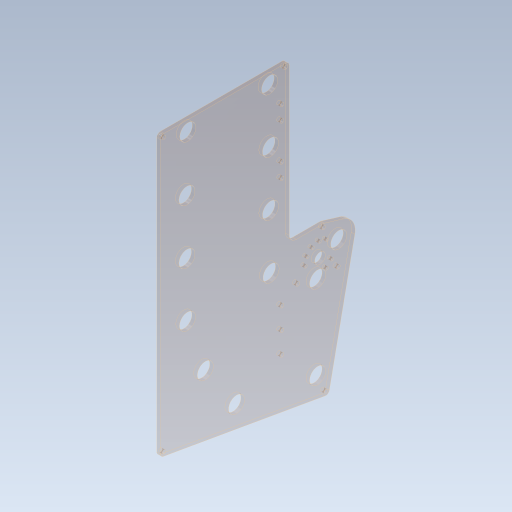
# Autodesk Inventor part: sketchers
Saved by Autodesk Inventor 2024 (Build 280153000, 153)
## iProperties
Created: 2024-07-27
Part Number: sketchers
Material: Polycarbonate, Smoke
Document SubType Name: Modeling
Designer: Oscar
Density: 1.2 g/cm^3
Appearance: Polycarbonate - Smoked
Author: Oscar
Autodesk Inventor part; units mm, degrees
ref_plane "YZ Plane" through (0, 0, 0) normal (1, 0, 0) x (0, 1, 0)
ref_plane "XZ Plane" through (0, 0, 0) normal (0, 1, 0) x (-1, 0, 0)
ref_plane "XY Plane" through (0, 0, 0) normal (0, 0, 1) x (1, 0, 0)
sketch "Sketch1" plane through (0, 0, 0) normal (1, 0, 0) x (0, 1, 0)
  line L0 (95.25, 812.8) -> (44.45, 812.8) construction
  line L1 (44.45, 812.8) -> (44.45, 0) construction
  line L2 (44.45, 0) -> (95.25, 0) construction
  line L3 (95.25, 0) -> (95.25, 812.8) construction
  line L4 (95.25, 0) -> (44.45, 0) construction
  line L5 (44.45, 0) -> (44.45, 25.4) construction
  line L6 (44.45, 25.4) -> (95.25, 25.4) construction
  line L7 (95.25, 25.4) -> (95.25, 0) construction
  circle A0 centre (190.5, 0) radius 50.8 construction
  circle A1 centre (95.25, 279.4) radius 25.4 construction
  circle A2 centre (274.6634, 275.1936) radius 9.525
  circle A3 centre (274.6634, 275.1936) radius 25.4 construction
  circle A4 centre (274.6634, 275.1936) radius 31.75 construction
  circle A5 centre (300.0634, 275.1936) radius 2.4892
  circle A6 centre (296.6604, 287.8936) radius 2.4892
  circle A7 centre (287.3634, 297.1907) radius 2.4892
  circle A8 centre (274.6634, 300.5936) radius 2.4892
  circle A9 centre (261.9634, 297.1907) radius 2.4892 construction
  circle A10 centre (252.6663, 287.8936) radius 2.4892 construction
  circle A11 centre (249.2634, 275.1936) radius 2.4892 construction
  circle A12 centre (252.6663, 262.4936) radius 2.4892
  circle A13 centre (261.9634, 253.1966) radius 2.4892
  circle A14 centre (274.6634, 249.7936) radius 2.4892 construction
  circle A15 centre (287.3634, 253.1966) radius 2.4892 construction
  circle A16 centre (296.6604, 262.4936) radius 2.4892
  circle A17 centre (609.6, 438.15) radius 50.8 construction
  circle A18 centre (274.6634, 275.1936) radius 30.48 construction
  circle A19 centre (587.8333, 365.125) radius 25.4 construction
  circle A20 centre (587.8333, 511.175) radius 25.4 construction
  line L8 (587.8333, 485.775) -> (587.8333, 390.525) construction
  circle A21 centre (490.3356, 512.7625) radius 14.351
  circle A22 centre (392.825, 512.7625) radius 14.351
  circle A23 centre (490.3356, 363.5375) radius 14.351
  line L9 (587.8333, 511.175) -> (490.3356, 512.7625) construction
  line L10 (587.8333, 365.125) -> (490.3356, 363.5375) construction
  circle A24 centre (490.3356, 512.7625) radius 25.4 construction
  circle A25 centre (490.3356, 363.5375) radius 25.4 construction
  line L11 (490.3356, 487.3625) -> (490.3356, 388.9375) construction
  circle A26 centre (392.825, 512.7625) radius 25.4 construction
  circle A27 centre (392.825, 363.5375) radius 25.4 construction
  circle A28 centre (392.825, 363.5375) radius 14.351
  line L12 (490.3356, 512.7625) -> (392.825, 512.7625) construction
  line L13 (490.3356, 363.5375) -> (392.825, 363.5375) construction
  line L14 (392.825, 487.3625) -> (392.825, 388.9375) construction
  circle A29 centre (295.3189, 511.8309) radius 25.4 construction
  circle A30 centre (295.3189, 362.6059) radius 25.4 construction
  circle A31 centre (203.1597, 479.9719) radius 25.4 construction
  circle A32 centre (295.3189, 511.8309) radius 14.351
  circle A33 centre (295.3189, 362.6059) radius 14.351
  circle A34 centre (203.1597, 479.9719) radius 14.351
  line L15 (392.825, 512.7625) -> (295.3189, 511.8309) construction
  line L16 (392.825, 363.5375) -> (295.3189, 362.6059) construction
  line L17 (295.3189, 486.4309) -> (295.3189, 388.0059) construction
  line L18 (295.3189, 511.8309) -> (203.1597, 479.9719) construction
  circle A35 centre (123.1487, 424.2353) radius 25.4 construction
  circle A36 centre (123.1487, 424.2353) radius 14.351
  line L19 (203.1597, 479.9719) -> (123.1487, 424.2353) construction
  circle A37 centre (95.25, 279.4) radius 14.351
  line L20 (609.6, 355.6) -> (44.45, 355.6) construction
  line L21 (44.45, 355.6) -> (44.45, 330.2) construction
  line L22 (44.45, 330.2) -> (609.6, 330.2) construction
  line L23 (609.6, 330.2) -> (609.6, 355.6) construction
  line L24 (95.25, 241.3) -> (44.45, 241.3) construction
  line L25 (44.45, 241.3) -> (44.45, 215.9) construction
  line L26 (44.45, 215.9) -> (95.25, 215.9) construction
  line L27 (95.25, 215.9) -> (95.25, 241.3) construction
  circle A38 centre (244.475, 279.4) radius 25.4 construction
  circle A39 centre (244.475, 279.4) radius 14.351
  line L28 (218.8463, 459.9947) -> (279.6322, 382.5831) construction
  circle A40 centre (274.6634, 275.1936) radius 8.89 construction
  circle A41 centre (286.5635, 241.6839) radius 26.67 construction
  circle A42 centre (244.475, 279.4) radius 21.59 construction
  circle A43 centre (286.5635, 241.6839) radius 14.351
  circle A44 centre (587.8333, 511.175) radius 14.351
  circle A45 centre (587.8333, 365.125) radius 14.351
  line L29 (44.45, 624.136) -> (44.45, 649.536) construction
  line L30 (95.25, 647.7) -> (609.6, 647.7) construction
  line L31 (609.6, 647.7) -> (609.6, 622.3) construction
  line L32 (609.6, 622.3) -> (95.25, 622.3) construction
  line L33 (95.25, 622.3) -> (95.25, 647.7) construction
  circle A46 centre (600.5333, 553.7721) radius 3.2639
  circle A47 centre (600.5333, 553.7721) radius 6.35 construction
  circle A48 centre (600.5333, 336.55) radius 3.2639
  circle A49 centre (600.5333, 336.55) radius 6.35 construction
  circle A50 centre (114.3, 553.7721) radius 3.2639
  circle A51 centre (114.3, 553.7721) radius 6.35 construction
  line L34 (595.0904, 535.5162) -> (598.719, 547.6868) construction
  circle A52 centre (63.5, 264.8503) radius 3.2639
  circle A53 centre (63.5, 264.8503) radius 6.35 construction
  line L35 (337.6816, 330.2) -> (600.5333, 330.2)
  line L36 (313.4556, 344.8233) -> (322.5239, 335.932) construction
  circle A54 centre (286.5635, 241.6839) radius 29.21 construction
  circle A55 centre (244.475, 279.4) radius 24.13 construction
  line L37 (72.1591, 268.8184) -> (69.2727, 267.4957) construction
  line L38 (609.6, 342.9) -> (44.45, 342.9) construction
  circle A56 centre (286.5635, 241.6839) radius 19.05 construction
  line L39 (262.4454, 263.2965) -> (264.8099, 261.1776) construction
  circle A57 centre (318.6316, 268.667) radius 3.2639
  circle A58 centre (254.5405, 314.8279) radius 3.2639
  circle A59 centre (244.6596, 242.3976) radius 3.2639
  line L40 (95.25, 558.8) -> (44.45, 558.8) construction
  line L41 (44.45, 558.8) -> (44.45, 533.4) construction
  line L42 (44.45, 533.4) -> (95.25, 533.4) construction
  line L43 (95.25, 533.4) -> (95.25, 558.8) construction
  line L44 (114.3, 560.1221) -> (600.5333, 560.1221)
  line L45 (108.0459, 554.8717) -> (57.2459, 265.95)
  line L46 (280.6003, 213.0891) -> (62.2036, 258.6341)
  circle A60 centre (318.6316, 268.667) radius 6.35 construction
  circle A61 centre (254.5405, 314.8279) radius 6.35 construction
  circle A62 centre (244.6596, 242.3976) radius 6.35 construction
  arc A63 (114.3, 560.1221) -> (108.0459, 554.8717) centre (114.3, 553.7721) ccw
  arc A64 (57.2459, 265.95) -> (62.2036, 258.6341) centre (63.5, 264.8503) ccw
  line L47 (312.3504, 269.5994) -> (306.0692, 270.5317) construction
  line L48 (313.7728, 264.5787) -> (308.914, 260.4903) construction
  line L49 (257.4152, 309.1658) -> (260.2899, 303.5038) construction
  line L50 (252.8051, 308.7196) -> (251.0697, 302.6114) construction
  line L51 (251.0087, 242.2895) -> (257.3577, 242.1814) construction
  line L52 (248.9458, 247.0828) -> (253.2321, 251.7679) construction
  line L53 (324.9816, 317.5) -> (324.9816, 268.667)
  arc A65 (337.6816, 330.2) -> (324.9816, 317.5) centre (337.6816, 317.5) ccw
  line L54 (324.7085, 266.8246) -> (314.5171, 233.2091)
  arc A66 (324.7085, 266.8246) -> (324.9816, 268.667) centre (318.6316, 268.667) ccw
  arc A67 (280.6003, 213.0891) -> (314.5171, 233.2091) centre (286.5635, 241.6839) ccw
  circle A68 centre (431.8, 342.9) radius 3.2639
  circle A69 centre (457.2, 342.9) radius 3.2639
  circle A70 centre (234.95, 342.9) radius 3.2639
  circle A71 centre (196.85, 342.9) radius 3.2639
  circle A72 centre (158.75, 342.9) radius 3.2639
  circle A73 centre (520.7, 342.9) radius 3.2639
  circle A74 centre (546.1, 342.9) radius 3.2639
  line L55 (606.8833, 553.7721) -> (606.8833, 336.55)
  arc A75 (606.8833, 553.7721) -> (600.5333, 560.1221) centre (600.5333, 553.7721) ccw
  arc A76 (600.5333, 330.2) -> (606.8833, 336.55) centre (600.5333, 336.55) ccw
  point P0 (0, 0)
  point P1 (273.4883, 247.5992)
  point P2 (276.276, 251.6898)
  point P3 (251.6966, 266.9984)
  point P4 (254.3358, 268.9733)
  dimension "d9" = 50.8
  dimension "d14" = 50.8
  dimension "d38" = 50.8
  dimension "d53" = 50.8
  dimension "d1" = 812.8
  dimension "d2" = 44.45
  dimension "d4" = 25.4
  dimension "d5" = 101.6
  dimension "d6" = 95.25
  dimension "d8" = 50.8
  dimension "d15" = 63.5
  dimension "d21" = 19.05
  dimension "d26" = 360
  dimension "d28" = 4.9784
  dimension "d29" = 438.15
  dimension "d30" = 514.35
  dimension "d36" = 60.96
  dimension "d39" = 50.8
  dimension "d41" = 95.25
  dimension "d45" = 28.702
  dimension "d47" = 97.5106
  dimension "d48" = 98.425
  dimension "d56" = 25.4
  dimension "d73" = 50.8
  dimension "d74" = 25.4
  dimension "d75" = 215.9
  dimension "d78" = 279.4
  dimension "d80" = 149.225
  dimension "d81" = 97.5106
  dimension "d82" = 147.4978
  dimension "d83" = 17.78
  dimension "d85" = 53.34
  dimension "d92" = 330.2
  dimension "d100" = 514.35
  dimension "d107" = 25.4
  dimension "d108" = 514.35
  dimension "d109" = 266.7
  dimension "d110" = 12.7
  dimension "d115" = 6.5278
  dimension "d116" = 12.7
  dimension "d122" = 2.54
  dimension "d123" = 2.54
  dimension "d128" = 3.175
  dimension "d133" = 38.1
  dimension "d134" = 3.175
  dimension "d135" = 194.9958
  dimension "d136" = 6.5278
  dimension "d137" = 25.4
  dimension "d138" = 533.4
  dimension "d139" = 19.05
  dimension "d140" = 19.05
  dimension "d141" = 12.7
  dimension "d142" = 6.35
  dimension "d143" = 12.7
  dimension "d144" = 43.18
  dimension "d149" = 25.4
  dimension "d151" = 6.5278
  dimension "d152" = 38.1
  dimension "d153" = 38.1
  dimension "d155" = 63.5
  dimension "d156" = 196.85
  dimension "d157" = 25.4
  dimension "d158" = 63.5
  dimension "d159" = 12.7
  constraints: 108 end point, 68 centre point, 47 point on circle, 32 point on line, 29 equal radius, 27 coincident, 20 tangent, 15 equal length, 11 parallel, 9 horizontal, 8 vertical alignment, 6 horizontal alignment, 6 perpendicular, 4 concentric, 4 vertical, 2 midpoint, 66 other
  measures "d1" distance of L1.end L0.end
  measures "d2" distance from line of point (0, 0) L1
  measures "d4" distance of L4.end L5.end
  measures "d5" diameter of A0
  measures "d15" diameter of A4
  measures "d21" diameter of A2
  measures "d28" diameter of A16
  measures "d29" distance from line of L2 point (609.6, 438.15)
  measures "d36" diameter of A18
  measures "d39" diameter of A20
  measures "d41" distance of L8.start L8.end
  measures "d45" diameter of A21
  measures "d47" distance of L9.start L9.end
  measures "d48" distance of L11.start L11.end
  measures "d56" distance of L22.end L20.start
  measures "d73" distance of L26.end L25.end
  measures "d74" distance of L25.end L24.end
  measures "d75" distance between parallel lines of L2 L26
  measures "d78" distance from line of L2 point (95.25, 279.4)
  measures "d80" distance of point (95.25, 279.4) A38.centre
  measures "d81" distance of A38.centre A30.centre
  measures "d82" distance of point (95.25, 279.4) A35.centre
  measures "d83" diameter of A40
  measures "d85" diameter of A41
  measures "d92" distance between parallel lines of L2 L22
  measures "d107" distance between parallel lines of L32 L30
  measures "d108" distance of L31.end L32.end
  measures "d109" distance between parallel lines of L20 L32
  measures "d110" distance of L34.start L34.end
  measures "d115" diameter of A46
  measures "d116" diameter of A47
  measures "d122" radial gap between concentric circles of A41 A54
  measures "d123" radial gap between concentric circles of A42 A55
  measures "d128" distance of L37.start L37.end
  measures "d133" diameter of A56
  measures "d134" distance of L39.start L39.end
  measures "d135" distance of A37.centre A43.centre
  measures "d136" diameter of A59
  measures "d137" distance between parallel lines of L40 L42
  measures "d138" distance between parallel lines of L2 L42
  measures "d140" distance from line of L1 A52.centre
  measures "d141" diameter of A62
  measures "d142" distance of L48.start L48.end
  measures "d143" radius of A65
  measures "d144" diameter of A42
  measures "d149" distance of A68.centre A69.centre
  measures "d151" diameter of A68
  measures "d152" distance of A70.centre A71.centre
  measures "d153" distance of A71.centre A72.centre
  measures "d156" distance of A68.centre A70.centre
  measures "d157" distance of A74.centre A73.centre
  measures "d158" distance of A69.centre A73.centre
  measures "d159" horizontal distance of L9.start A47.centre
extrude "Extrusion2" add sketch "Sketch1" along normal blind 6.35
body "Solid2"
